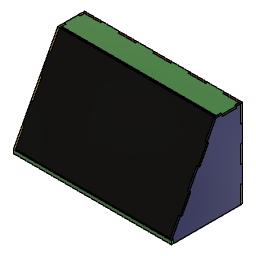
unsorted_smarties_holder_finger_joints (Autodesk Fusion 360 design; units mm, degrees)
Autodesk Fusion 360 part; units mm, degrees
note: some values were not read from the file. Chosen so that the rebuilt part matches the saved one: which bodies a step acts on; which face or edge a step refers to.
sketch "Unsorted Smarties Holder" plane through (0, 0, 0) normal (1, 0, 0) x (0, 1, 0)
  line L0 (0, 0) -> (92.371665, 0)
  line L1 (92.371665, 0) -> (92.371665, 142)
  line L2 (92.371665, 142) -> (47.371665, 142)
  line L3 (47.371665, 142) -> (-27.628335, 0)
  line L4 (-27.628335, 0) -> (0, 0)
  line L5 (-27.628335, 0) -> (92.371665, 0)
  line L6 (92.371665, 0) -> (92.371665, -6)
  line L7 (92.371665, -6) -> (-27.628335, -6)
  line L8 (-27.628335, -6) -> (-27.628335, 0)
  dimension "d5" = 142
  dimension "d23" = 120
  dimension "d31" = 6
  dimension "d34" = 45
  constraint horizontal L0
  constraint vertical L1
  constraint horizontal L2
  constraint coincident L0.start L4.end
  constraint horizontal L5
  constraint vertical L6
  constraint horizontal L7
  constraint vertical L8
  constraint collinear L1 L6
  measures "d31" distance of L0 L7
extrude "Extrude1" add sketch "Unsorted Smarties Holder" along normal blind 268 makes body 1
sketch "Chamber" plane through (268, 0, 0) normal (1, 0, 0) x (0, 1, 0)
  line L0 (92.371665, -6) -> (92.371665, 142)
  line L1 (92.371665, 142) -> (47.371665, 142)
  line L2 (47.371665, 142) -> (-27.628335, 0)
  line L3 (89.371665, 139) -> (89.371665, 0)
  line L4 (89.371665, 0) -> (-24.235599, 0)
  line L5 (-24.235599, 0) -> (49.179894, 139)
  line L6 (49.179894, 139) -> (89.371665, 139)
  line L7 (-27.628335, 0) -> (-27.628335, -6)
  line L8 (-27.628335, -6) -> (92.371665, -6)
  line L9 (-24.235599, 0) -> (89.371665, 0)
  line L10 (89.371665, 0) -> (89.371665, -6)
  line L11 (89.371665, -6) -> (-24.235599, -6)
  line L12 (-24.235599, -6) -> (-24.235599, 0)
  dimension "d15" = 3
  dimension "d16" = 3
  dimension "d17" = 3
  dimension "d18" = 3
  dimension "d32" = 6
  dimension "d33" = 6
  constraint perpendicular L1 L3
  constraint perpendicular L3 L4
  constraint parallel L2 L5
  constraint horizontal L9
  constraint vertical L10
  constraint horizontal L11
  constraint vertical L12
  constraint collinear L3 L10
  measures "d17" distance of L2 L5
  measures "d18" distance of L0 L3
  measures "d32" distance of L4 L8
  measures "d33" distance of L9 L11
extrude "Extrude3" cut sketch "Chamber" against normal blind 264 from surface at -3 contours L4 L8 L9 L10 L11 L12 | L3 L4 L5 L6 L9 picked at (51.502577, -2) picked at (38.10532, 46.333333) bodies 1
sketch "Smarties Feed" plane through (0, 92.371665, 0) normal (0, 1, 0) x (-1, 0, 0)
  line L0 (0, -6) -> (0, 142)
  line L1 (0, 142) -> (-268, 142)
  line L2 (-268, 142) -> (-268, -6)
  line L3 (-179, 107) -> (-89, 107)
  line L4 (-89, 107) -> (-89, 77)
  line L5 (-89, 77) -> (-179, 77)
  line L6 (-179, 77) -> (-179, 107)
  line L7 (-268, -6) -> (0, -6)
  dimension "d24" = 30
  dimension "d25" = 90
  dimension "d26" = 89
  dimension "d27" = 89
  dimension "d28" = 35
  constraint horizontal L3
  constraint vertical L4
  constraint horizontal L5
  constraint vertical L6
  measures "d24" distance of L3.end L4.end
  measures "d25" distance of L3.start L3.end
  measures "d26" distance of L2 L6
  measures "d27" distance of L0 L4
  measures "d28" distance of L1 L3
extrude "Extrude4" cut sketch "Smarties Feed" against normal blind 3 contours L3 L4 L5 L6 picked at (-119, 87) bodies 1
ref_plane "WorkPlane1" through (133, 89.371665, 66.5) normal (0, -1, 0) x (0, 0, 1)
ref_plane "WorkPlane2" through (265, 32.568033, 66.5) normal (-1, 0, 0) x (0, -1, 0)
ref_plane "WorkPlane3" through (1, 32.568033, 66.5) normal (1, 0, 0) x (0, 0, -1)
ref_plane "WorkPlane4" through (133, 12.472148, 69.5) normal (0, 0.884242, -0.467029) x (0, -0.467029, -0.884242)
ref_plane "WorkPlane5" through (133, -24.235599, -3) normal (0, 1, 0) x (0, 0, -1)
split "Split1" by plane through (133, 89.371665, 66.5) normal (0, -1, 0) bodies 1 makes body 2 at (178.666667, 22.371665, 94.666667)
move_body "Move1" bodies 1 to x (1, 0, 0) y (0, 1, 0) z (0, 0, 1) at (0, 80, 0)
split "Split2" by plane through (1, 32.568033, 66.5) normal (1, 0, 0) bodies 2 makes body 3 at (90, 22.371665, 94.666667)
move_body "Move2" bodies 2 to x (1, 0, 0) y (0, 1, 0) z (0, 0, 1) at (0, -80, 0)
split "Split3" by plane through (265, 32.568033, 66.5) normal (-1, 0, 0) bodies 3 makes body 4 at (89, 22.371665, 94.666667)
move_body "Move3" bodies 3 to x (1, 0, 0) y (0, 1, 0) z (0, 0, 1) at (80, 0, 0)
split "Split4" by plane through (133, 12.472148, 69.5) normal (0, 0.884242, -0.467029) bodies 4 makes body 5 at (177, 62.577151, 139) makes body 6 at (177, -24.235599, -4)
move_body "Move4" bodies 5 to x (1, 0, 0) y (0, 1, 0) z (0, 0, 1) at (0, 0, 80)
move_body "Move5" bodies 2 to x (1, 0, 0) y (0, 1, 0) z (0, 0, 1) at (-80, 80, 0)
combine "Combine1" operation add target body 6 tool bodies 4
ref_plane "WorkPlane6" through (133, -25.931967, 0) normal (0, 0, -1) x (0, 1, 0)
split "Split5" by plane through (133, -25.931967, 0) normal (0, 0, -1) bodies 6 makes body 7 at (89, -27.628335, -4)
move_body "Move6" bodies 7 to x (1, 0, 0) y (0, 1, 0) z (0, 0, 1) at (0, 0, -80)
move_body "Move7" bodies 2 to x (1, 0, 0) y (0, 1, 0) z (0, 0, 1) at (80, 0, 0)
move_body "Move8" bodies 1 to x (1, 0, 0) y (0, 1, 0) z (0, 0, 1) at (0, -80, 0)
move_body "Move9" bodies 3 to x (1, 0, 0) y (0, 1, 0) z (0, 0, 1) at (-80, 0, 0)
move_body "Move10" bodies 5 to x (1, 0, 0) y (0, 1, 0) z (0, 0, 1) at (0, 0, -80)
move_body "Move11" bodies 7 to x (1, 0, 0) y (0, 1, 0) z (0, 0, 1) at (0, 0, 0)
move_body "Move12" bodies 7 to x (1, 0, 0) y (0, 1, 0) z (0, 0, 1) at (0, 0, 160)
move_body "Move13" bodies 7 to x (1, 0, 0) y (0, 1, 0) z (0, 0, 1) at (0, 0, -80)
sketch "Sketch5" plane through (268, 0, 0) normal (1, 0, 0) x (0, 1, 0)
  line L0 (89.371665, -6) -> (89.371665, 142)
  line L1 (89.371665, 142) -> (47.371665, 142)
  line L2 (47.371665, 142) -> (-27.628335, 0)
  line L3 (-27.628335, 0) -> (-27.628335, -6)
  line L4 (-27.628335, -6) -> (89.371665, -6)
  line L5 (92.371665, -6) -> (92.371665, 142)
  line L6 (92.371665, 142) -> (89.371665, 142)
  line L7 (92.371665, 112.4) -> (89.371665, 112.4)
  line L8 (92.371665, -6) -> (89.371665, -6)
  line L9 (92.371665, 23.6) -> (89.371665, 23.6)
  line L10 (92.371665, 82.8) -> (89.371665, 82.8)
  line L11 (92.371665, 53.2) -> (89.371665, 53.2)
  dimension "d41" = 3
  dimension "d42" = -29.6
  dimension "d43" = 29.6
  dimension "d44" = -59.2
  dimension "d45" = 59.2
  constraint perpendicular L0 L6
  constraint perpendicular L0 L8
extrude "Extrude5" cut sketch "Sketch5" against normal blind 3 contours L0 L5 L9 L11 | L0 L5 L7 L10 picked at (90.371665, 33.466667) picked at (90.371665, 102.533333) bodies 1
extrude "Extrude6" add sketch "Sketch5" against normal blind 3 contours L0 L5 L9 L11 | L0 L5 L7 L10 picked at (90.371665, 33.466667) picked at (90.371665, 102.533333) bodies 3
sketch "Sketch6" plane through (0, -21.602146, 11.409584) normal (0, -0.884242, 0.467029) x (1, 0, 0)
  line L0 (265, -12.903239) -> (265, 147.6863)
  line L1 (265, 147.6863) -> (1, 147.6863)
  line L2 (1, 147.6863) -> (1, -12.903239)
  line L3 (1, -12.903239) -> (265, -12.903239)
  line L4 (268, -12.903239) -> (268, 147.6863)
  line L5 (265, 115.6863) -> (1, 115.6863)
  line L6 (265, 83.6863) -> (1, 83.6863)
  line L7 (1, 19.096761) -> (265, 19.096761)
  line L8 (1, 51.096761) -> (265, 51.096761)
  line L9 (265, 115.6863) -> (268, 115.6863)
  line L10 (265, 83.6863) -> (268, 83.6863)
  line L11 (265, 51.096761) -> (268, 51.096761)
  line L12 (268, 51.096761) -> (265, 51.096761)
  line L13 (265, 51.096761) -> (265, 19.096761)
  line L14 (265, 19.096761) -> (268, 19.096761)
  line L15 (268, 19.096761) -> (268, 51.096761)
  dimension "d50" = 3
  dimension "d51" = -32
  dimension "d52" = -64
  dimension "d53" = -32
  dimension "d54" = -64
  dimension "d55" = 3
  constraint coincident L4 L9.end
  constraint perpendicular L4 L9
  constraint coincident L4 L10.end
  constraint perpendicular L4 L10
  constraint perpendicular L0 L11
  constraint horizontal L12
  constraint vertical L13
  constraint horizontal L14
  constraint vertical L15
extrude "Extrude7" cut sketch "Sketch6" against normal blind 3 contours L0 L4 L11 L12 L13 L14 L15 | L0 L4 L9 L10 picked at (266, 40.430095) picked at (266, 94.352967) bodies 3
extrude "Extrude8" add sketch "Sketch6" against normal blind 3 separate body contours L0 L4 L11 L12 L13 L14 L15 | L0 L4 L9 L10 picked at (266, 40.430095) picked at (266, 94.352967) makes body 8 at (265, 29.21357, 103.338287) makes body 9 at (265, -6.817515, 37.260625)
combine "Combine2" operation add target body 6 tool bodies 8 9
sketch "Sketch7" plane through (0, 0, 142) normal (0, 0, 1) x (-1, 0, 0)
  line L0 (-1, -50.764401) -> (-265, -50.764401)
  line L1 (-265, -50.764401) -> (-265, -89.371665)
  line L2 (-265, -89.371665) -> (-1, -89.371665)
  line L3 (-1, -89.371665) -> (-1, -50.764401)
  line L4 (-268, -50.764401) -> (-268, -89.371665)
  line L5 (-265, -70.068033) -> (-265, -82.068033)
  line L6 (-265, -70.068033) -> (-268, -70.068033)
  line L7 (-268, -70.068033) -> (-268, -58.068033)
  line L8 (-265, -82.068033) -> (-268, -82.068033)
  line L9 (-268, -82.068033) -> (-268, -58.068033)
  line L10 (-268, -58.068033) -> (-265, -58.068033)
  line L11 (-265, -58.068033) -> (-265, -82.068033)
  dimension "d60" = 3
  dimension "d61" = 12
  dimension "d62" = 3
  dimension "d63" = 12
  constraint perpendicular L2 L5
  constraint perpendicular L1 L6
  constraint perpendicular L6 L7
  constraint horizontal L8
  constraint vertical L9
  constraint horizontal L10
  constraint vertical L11
extrude "Extrude9" cut sketch "Sketch7" against normal blind 3 contours L1 L4 L6 L7 L9 L10 L11 | L1 L4 L5 L6 L8 L9 L11 picked at (-266, -62.068033) picked at (-266, -78.068033) bodies 3
extrude "Extrude10" add sketch "Sketch7" against normal blind 3 separate body contours L1 L4 L6 L7 L9 L10 L11 | L1 L4 L5 L6 L8 L9 L11 picked at (-266, -62.068033) picked at (-266, -78.068033) makes body 10
combine "Combine3" operation add target body 5 tool bodies 10
delete_body "RemoveBody1" bodies 2
mirror "Mirror1" about plane through (0, 0, 0) normal (1, 0, 0) of bodies 3 makes body 11
move_body "Move14" bodies 11 to x (1, 0, 0) y (0, 1, 0) z (0, 0, 1) at (180, 0, 0)
move_body "Move15" bodies 11 to x (1, 0, 0) y (0, 1, 0) z (0, 0, 1) at (89, 0, 0)
extrude "Extrude11" cut 1 faces at (0, 90.371665, 43.333333) along direction (1, 0, 0) blind 1 on bodies 1 bodies 1
ref_plane "WorkPlane7" through (133, 11.198028, 70.299456) normal (1, 0, 0) x (0, 0, -1)
sketch "Sketch8" plane through (0, 92.371665, 0) normal (0, 1, 0) x (-1, 0, 0)
  line L0 (-1, -6) -> (-1, 142)
  line L1 (-1, 142) -> (-268, 142)
  line L2 (-268, 142) -> (-268, 112.4)
  line L3 (-268, 112.4) -> (-265, 112.4)
  line L4 (-265, 112.4) -> (-265, 82.8)
  line L5 (-265, 82.8) -> (-268, 82.8)
  line L6 (-268, 82.8) -> (-268, 53.2)
  line L7 (-268, 53.2) -> (-265, 53.2)
  line L8 (-265, 53.2) -> (-265, 23.6)
  line L9 (-265, 23.6) -> (-268, 23.6)
  line L10 (-268, 23.6) -> (-268, -6)
  line L11 (-268, -6) -> (-1, -6)
  line L12 (-89, 107) -> (-89, 77)
  line L13 (-89, 77) -> (-179, 77)
  line L14 (-179, 77) -> (-179, 107)
  line L15 (-179, 107) -> (-89, 107)
  line L16 (-4, -6) -> (-4, 142)
  line L17 (-265, 112.4) -> (132.111416, 112.4)
  line L18 (-265, 23.6) -> (146.671472, 23.6)
  line L19 (-265, 82.8) -> (163.303646, 82.8)
  line L20 (-265, 53.2) -> (137.265795, 53.2)
  dimension "d72" = -3
  constraint coincident L3.end L4.start
  constraint perpendicular L0 L17
  constraint coincident L8.end L9.start
  constraint perpendicular L8 L18
  constraint coincident L4.end L5.start
  constraint perpendicular L4 L19
  constraint coincident L7.end L8.start
  constraint perpendicular L8 L20
extrude "Extrude12" cut sketch "Sketch8" against normal blind 5 contours L0 L16 L18 L20 | L0 L16 L17 L19 picked at (-2, 33.466667) picked at (-3, 92.666667) bodies 1
sketch "Sketch9" plane through (0, 0, 142) normal (0, 0, 1) x (-1, 0, 0)
  line L0 (-1, -50.764401) -> (-265, -50.764401)
  line L1 (-265, -50.764401) -> (-265, -58.068033)
  line L2 (-265, -58.068033) -> (-268, -58.068033)
  line L3 (-268, -58.068033) -> (-268, -82.068033)
  line L4 (-268, -82.068033) -> (-265, -82.068033)
  line L5 (-265, -82.068033) -> (-265, -89.371665)
  line L6 (-265, -89.371665) -> (-1, -89.371665)
  line L7 (-1, -89.371665) -> (-1, -50.764401)
  line L8 (-1, -58.068033) -> (-4, -58.068033)
  line L9 (-4, -58.068033) -> (-4, -50.764401)
  line L10 (-4, -89.371665) -> (-4, -82.068033)
  line L11 (-4, -82.068033) -> (-1, -82.068033)
  line L12 (-4, -89.371665) -> (-1, -89.371665)
  line L13 (-1, -89.371665) -> (-1, -82.068033)
  line L14 (-1, -82.068033) -> (-4, -82.068033)
  line L15 (-4, -82.068033) -> (-4, -89.371665)
  line L16 (-1, -58.068033) -> (-4, -58.068033)
  line L17 (-4, -58.068033) -> (-4, -50.764401)
  line L18 (-4, -50.764401) -> (-1, -50.764401)
  line L19 (-1, -50.764401) -> (-1, -58.068033)
  point P0 (-1, -58.068033)
  point P1 (-4, -58.068033)
  point P2 (-4, -89.371665)
  point P3 (-4, -82.068033)
  dimension "d75" = 3
  constraint perpendicular L0 L9
  constraint perpendicular L7 L11
  constraint horizontal L12
  constraint vertical L13
  constraint horizontal L14
  constraint vertical L15
  constraint horizontal L16
  constraint vertical L17
  constraint horizontal L18
  constraint vertical L19
extrude "Extrude13" cut sketch "Sketch9" against normal blind 8 contours L0 L7 L8 L9 L16 L17 L18 L19 | L6 L7 L10 L11 L12 L13 L14 L15 picked at (-2, -55.633489) picked at (-2, -86.937121) bodies 5
sketch "Sketch10" plane through (0, -21.602146, 11.409584) normal (0, -0.884242, 0.467029) x (1, 0, 0)
  line L0 (265, -12.903239) -> (265, 19.096761)
  line L1 (265, 19.096761) -> (268, 19.096761)
  line L2 (268, 19.096761) -> (268, 51.096761)
  line L3 (268, 51.096761) -> (265, 51.096761)
  line L4 (265, 51.096761) -> (265, 83.6863)
  line L5 (265, 83.6863) -> (268, 83.6863)
  line L6 (268, 83.6863) -> (268, 115.6863)
  line L7 (268, 115.6863) -> (265, 115.6863)
  line L8 (265, 115.6863) -> (265, 147.6863)
  line L9 (265, 147.6863) -> (1, 147.6863)
  line L10 (1, 147.6863) -> (1, -12.903239)
  line L11 (1, -12.903239) -> (265, -12.903239)
  line L12 (1, 147.6863) -> (4, 147.6863)
  line L13 (4, 147.6863) -> (4, 115.6863)
  line L14 (4, 115.6863) -> (1, 115.6863)
  line L15 (1, 115.6863) -> (1, 147.6863)
  line L16 (1, 83.6863) -> (4, 83.6863)
  line L17 (4, 83.6863) -> (4, 51.096761)
  line L18 (4, 51.096761) -> (1, 51.096761)
  line L19 (1, 51.096761) -> (1, 83.6863)
  line L20 (1, 19.096761) -> (4, 19.096761)
  line L21 (4, 19.096761) -> (4, -12.903239)
  line L22 (4, -12.903239) -> (1, -12.903239)
  line L23 (1, -12.903239) -> (1, 19.096761)
  line L24 (4, 115.6863) -> (1, 115.6863)
  line L25 (1, 115.6863) -> (1, 83.6863)
  line L26 (1, 83.6863) -> (4, 83.6863)
  line L27 (4, 83.6863) -> (4, 115.6863)
  line L28 (4, 51.096761) -> (1, 51.096761)
  line L29 (1, 51.096761) -> (1, 19.096761)
  line L30 (1, 19.096761) -> (4, 19.096761)
  line L31 (4, 19.096761) -> (4, 51.096761)
  point P0 (4, 115.6863)
  point P1 (1, 83.6863)
  point P2 (4, 51.096761)
  point P3 (1, 19.096761)
  point P4 (4, -12.903239)
  constraint horizontal L12
  constraint vertical L13
  constraint horizontal L14
  constraint vertical L15
  constraint coincident P0 L13.end
  constraint coincident L9.end L10.start
  constraint horizontal L16
  constraint vertical L17
  constraint horizontal L18
  constraint vertical L19
  constraint coincident P1 L16.start
  constraint horizontal L20
  constraint vertical L21
  constraint horizontal L22
  constraint vertical L23
  constraint horizontal L24
  constraint vertical L25
  constraint horizontal L26
  constraint vertical L27
  constraint horizontal L28
  constraint vertical L29
  constraint horizontal L30
  constraint vertical L31
extrude "Extrude14" cut sketch "Sketch10" against normal blind 20 contours L10 L11 L20 L21 L22 L23 L30 | L10 L16 L17 L18 L19 L26 L28 | L9 L10 L12 L13 L14 L15 L24 picked at (2, 8.430095) picked at (3, 61.959941) picked at (3, 137.019634) bodies 6 7
extrude "Extrude15" cut 1 faces at (2, 49.140149, 141.065942) along direction (0, 0.46702918, 0.88424191) blind 3 on bodies 6 bodies 6
extrude "Extrude16" cut 1 faces at (1, 50.236232, 140) along direction (1, 0, 0) blind 3 on bodies 5 bodies 5
extrude "Extrude17" cut 1 faces at (1, -26.497423, -2.597313) along direction (1, 0, 0) blind 3 on bodies 7 bodies 7
sketch "Sketch11" plane through (4, 0, 0) normal (-1, 0, 0) x (0, -1, 0)
  line L0 (-58.068033, 139) -> (-49.179894, 139)
  line L1 (-49.179894, 139) -> (-50.764401, 142)
  line L2 (-50.764401, 142) -> (-58.068033, 142)
  line L3 (-58.068033, 142) -> (-58.068033, 139)
  line L4 (-50.764401, 142) -> (-50.764401, 139.005692)
  line L5 (-50.764401, 142) -> (-49.179894, 139)
  line L6 (-50.764401, 139.005692) -> (-49.179894, 139)
  point P0 (-50.764401, 142)
  constraint vertical L4
extrude "Extrude18" cut sketch "Sketch11" against normal blind 290 contours L1 L4 L5 L6 picked at (-50.236232, 140.001897) bodies 5
extrude "Extrude19" cut 1 faces at (91, 50.236232, 139.003795) along direction (0, 0.00359258, -0.99999355) blind 3 on bodies 5 bodies 5
move_body "Move16" bodies 6 to x (1, 0, 0) y (0, 1, 0) z (0, 0, 1) at (0, -60, 0)
move_body "Align1" bodies 6 to x (1, 0, 0) y (0, 0.88424191, 0.46702918) z (0, -0.46702918, 0.88424191) at (0, 166.856311, 27.045713)
move_body "Move17" bodies 6 to x (1, 0, 0) y (0, 1, 0) z (0, 0, 1) at (0, 0, 160)
sketch "Sketch12" plane through (265, 0, 0) normal (1, 0, 0) x (0, 1, 0)
  line L0 (89.371665, 274.710262) -> (92.371665, 274.710262)
  line L1 (92.371665, 274.710262) -> (92.371665, 308.294769)
  line L2 (92.371665, 308.294769) -> (89.371665, 306.710262)
  line L3 (89.371665, 306.710262) -> (89.371665, 274.710262)
  line L4 (89.371665, 306.710262) -> (97.803432, 306.710262)
  constraint perpendicular L3 L4
extrude "Extrude20" cut sketch "Sketch12" against normal blind 320 contours L1 L2 L4 picked at (91.371665, 307.238431) bodies 6
sketch "Sketch13" plane through (265, 0, 0) normal (1, 0, 0) x (0, 1, 0)
  line L0 (92.371665, 178.120724) -> (89.371665, 178.120724)
  line L1 (89.371665, 178.120724) -> (89.371665, 146.120724)
  line L2 (89.371665, 146.120724) -> (92.371665, 147.705231)
  line L3 (92.371665, 147.705231) -> (92.371665, 178.120724)
  line L4 (92.371665, 147.705231) -> (82.776425, 147.465847)
extrude "Extrude21" cut sketch "Sketch13" against normal blind 310 contours L1 L2 L4 picked at (90.371665, 147.152113) bodies 6
move_body "Align2" bodies 6 to x (1, 0, 0) y (0, 0.88424191, -0.46702918) z (0, 0.46702918, 0.88424191) at (0, -174.897148, -87.466892)
sketch "Sketch14" plane through (0, 0, 142) normal (0, 0, 1) x (-1, 0, 0)
  line L0 (-4, -82.068033) -> (-1, -82.068033)
  line L1 (-1, -82.068033) -> (-1, -58.068033)
  line L2 (-1, -58.068033) -> (-4, -58.068033)
  line L3 (-4, -58.068033) -> (-4, -50.764401)
  line L4 (-4, -50.764401) -> (-265, -50.764401)
  line L5 (-265, -50.764401) -> (-265, -58.068033)
  line L6 (-265, -58.068033) -> (-268, -58.068033)
  line L7 (-268, -58.068033) -> (-268, -82.068033)
  line L8 (-268, -82.068033) -> (-265, -82.068033)
  line L9 (-265, -82.068033) -> (-265, -89.371665)
  line L10 (-265, -89.371665) -> (-4, -89.371665)
  line L11 (-4, -89.371665) -> (-4, -82.068033)
  line L12 (-134.5, -89.371665) -> (-134.5, 52.227808)
  line L13 (-134.5, -89.371665) -> (-119.7, -89.371665)
  line L14 (-134.5, -89.371665) -> (-149.3, -89.371665)
  line L15 (-119.7, -89.371665) -> (-90.1, -89.371665)
  line L16 (-149.3, -89.371665) -> (-178.9, -89.371665)
  line L17 (-90.1, -89.371665) -> (-60.5, -89.371665)
  line L18 (-60.5, -89.371665) -> (-30.9, -89.371665)
  line L19 (-178.9, -89.371665) -> (-208.5, -89.371665)
  line L20 (-208.5, -89.371665) -> (-238.1, -89.371665)
  line L21 (-30.9, -89.371665) -> (-30.9, -92.371665)
  line L22 (-60.5, -89.371665) -> (-30.9, -89.371665)
  line L23 (-30.9, -89.371665) -> (-30.9, -92.371665)
  line L24 (-30.9, -92.371665) -> (-60.5, -92.371665)
  line L25 (-60.5, -92.371665) -> (-60.5, -89.371665)
  line L26 (-90.1, -89.371665) -> (-90.1, -92.371665)
  line L27 (-119.7, -89.371665) -> (-90.1, -89.371665)
  line L28 (-90.1, -89.371665) -> (-90.1, -92.371665)
  line L29 (-90.1, -92.371665) -> (-119.7, -92.371665)
  line L30 (-119.7, -92.371665) -> (-119.7, -89.371665)
  line L31 (-238.1, -89.371665) -> (-238.1, -92.371665)
  line L32 (-238.1, -92.371665) -> (-208.5, -92.371665)
  line L33 (-208.5, -92.371665) -> (-208.5, -89.371665)
  line L34 (-208.5, -89.371665) -> (-238.1, -89.371665)
  line L35 (-238.1, -89.371665) -> (-238.1, -92.371665)
  line L36 (-178.9, -89.371665) -> (-178.9, -92.371665)
  line L37 (-178.9, -92.371665) -> (-149.3, -92.371665)
  line L38 (-149.3, -92.371665) -> (-178.9, -92.371665)
  line L39 (-178.9, -92.371665) -> (-178.9, -89.371665)
  line L40 (-178.9, -89.371665) -> (-149.3, -89.371665)
  line L41 (-149.3, -89.371665) -> (-149.3, -92.371665)
  dimension "d94" = 14.8
  dimension "d95" = 14.8
  dimension "d96" = 29.6
  dimension "d97" = 29.6
  dimension "d98" = 29.6
  dimension "d99" = 29.6
  dimension "d100" = 29.6
  dimension "d101" = 29.6
  dimension "d102" = 3
  dimension "d103" = 3
  dimension "d104" = 3
  dimension "d105" = 3
  dimension "d106" = 29.6
  constraint perpendicular L4 L12
  constraint perpendicular L12 L13
  constraint perpendicular L12 L14
  constraint parallel L10 L15
  constraint perpendicular L7 L16
  constraint parallel L10 L17
  constraint perpendicular L11 L18
  constraint parallel L16 L19
  constraint parallel L10 L20
  constraint perpendicular L18 L21
  constraint horizontal L22
  constraint vertical L23
  constraint horizontal L24
  constraint vertical L25
  constraint perpendicular L17 L26
  constraint horizontal L27
  constraint vertical L28
  constraint horizontal L29
  constraint vertical L30
  constraint perpendicular L20 L31
  constraint horizontal L32
  constraint vertical L33
  constraint horizontal L34
  constraint vertical L35
  constraint perpendicular L19 L36
  constraint perpendicular L36 L37
  constraint horizontal L38
  constraint vertical L39
  constraint horizontal L40
  constraint vertical L41
extrude "Extrude22" cut sketch "Sketch14" against normal blind 3 contours L10 L18 L21 L22 L23 L24 L25 | L10 L15 L26 L27 L28 L29 L30 | L10 L16 L36 L37 L38 L39 L40 L41 | L10 L20 L31 L32 L33 L34 L35 picked at (-40.766667, -91.371665) picked at (-109.833333, -91.371665) picked at (-169.033333, -90.371665) picked at (-228.233333, -90.371665) bodies 1
extrude "Extrude23" add 4 faces at (40.766667, 91.371665, 139) (109.833333, 91.371665, 139) (169.033333, 90.371665, 139) (228.233333, 90.371665, 139) along direction (0, 0, 1) blind 3 separate body on bodies 1 makes body 12 at (169.033333, 90.371665, 139) makes body 13 at (50.633333, 89.371665, 140) makes body 14 at (109.833333, 91.371665, 139) makes body 15 at (228.233333, 90.371665, 139)
combine "Combine4" operation add target body 5 tool bodies 12 13 14 15
extrude "Extrude24" cut 1 faces at (265, -26.497423, -2) along direction (1, 0, 0) blind 3 on bodies 7 bodies 3
extrude "Extrude25" cut 1 faces at (4, -26.497423, -2) along direction (-1, 0, 0) blind 3 on bodies 7 bodies 11
extrude "Extrude26" add 1 faces at (265, -26.497423, -2) along direction (1, 0, 0) blind 3 on bodies 7 bodies 7
extrude "Extrude27" add 1 faces at (4, -26.497423, -2) along direction (-1, 0, 0) blind 3 on bodies 7 bodies 7
equation "polycarbonateThickness = 3 mm" comment "Thickness of the polycarbonate panels"
equation "d15 = polycarbonateThickness"
equation "d16 = polycarbonateThickness"
equation "d17 = polycarbonateThickness"
equation "d18 = polycarbonateThickness"
equation "d20 = -polycarbonateThickness"
equation "d21 = -( 270 mm - 2 * polycarbonateThickness )"
equation "d28 = 41 mm - 6 mm"
equation "d29 = -polycarbonateThickness"
named bodies: "Unsorted Smarties Holder", "Unsorted Smarties Holder (1)", "Unsorted Smarties Holder (1) (1)", "Unsorted Smarties Holder (1) (1) (1)", "Unsorted Smarties Holder (1) (1) (1) (1)", "Unsorted Smarties Holder (1) (1) (1) (2)", "Unsorted Smarties Holder (1) (1) (1) (2) (1)"
